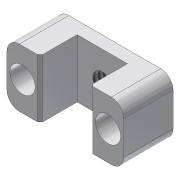
# Autodesk Inventor part: J002866
Saved by Autodesk Inventor 2012 SP2 (Build 160219200, 219)
## iProperties
Created: 2014-09-05
Material: ALUMINUM, 6061-T651
Vendor: HHMI: JFRC - ID&F
Document SubType Name: Modeling
Designer: arnoldj
Density: 2.7 g/cm^3
Part Number: J002866
Description: MPS Clamp Base
Mass: 8.49336 g
Surface Area: 23.5397 cm^2
Volume: 3.14569 cm^3
Project: P-194005
RuleStatus: InUse
AfterDocSave0: file://Part Number Cleaner
LAB/DEPT: SVOBODA (LAB)
REQUESTING SCIENTIST: PERON, SIMON
SURFACE ROUGHNESS: 63 Ra
DESIGN DEPARTMENT: HHMI: JFRC - ID&F
SPECIAL FINISH: ANODIZE PER MIL-A-8625F, TYPE II, CLASS 2 (BLACK)
ALTERED ITEM PART NUMBER: N/A
ALTERED ITEM VENDOR: N/A
ALTERED ITEM DESCRIPTION: N/A
PART NUMBER - LEGACY: J002866
Revision Number: -
Autodesk Inventor part; units mm, degrees
ref_plane "YZ Plane" through (0, 0, 0) normal (1, 0, 0) x (0, 1, 0)
ref_plane "XZ Plane" through (0, 0, 0) normal (0, 1, 0) x (-1, 0, 0)
ref_plane "XY Plane" through (0, 0, 0) normal (0, 0, 1) x (1, 0, 0)
sketch "Sketch1" plane through (0, 0, 0) normal (0, 0, 1) x (1, 0, 0)
  line L0 (-15, 7.5) -> (15, 7.5)
  line L1 (15, 7.5) -> (15, -7.5)
  line L2 (15, -7.5) -> (-15, -7.5)
  line L3 (-15, -7.5) -> (-15, 7.5)
  point P0 (0, 0)
  point P1 (-15, 0)
  point P2 (0, 7.5)
  dimension "d0" = 30
  dimension "d1" = 15
  constraints: 8 end point, 2 midpoint, 2 parallel, 1 horizontal, 1 horizontal alignment, 1 perpendicular, 1 vertical alignment
  measures "d0" distance of L0.start L0.end
  measures "d1" distance of L0.end L1.end
extrude "Extrusion1" add sketch "Sketch1" along normal blind 12.7
sketch "Sketch3" plane through (0, 0, 12.7) normal (0, 0, 1) x (1, 0, 0)
  line L0 (-15, 7.5) -> (15, 7.5) projected
  line L1 (15, -7.5) -> (-15, -7.5) projected
  line L2 (-6.477, 7.5) -> (6.477, 7.5)
  line L3 (6.477, 7.5) -> (6.477, -7.5)
  line L4 (6.477, -7.5) -> (-6.477, -7.5)
  line L5 (-6.477, -7.5) -> (-6.477, 7.5)
  point P0 (0, 0)
  point P1 (0, 7.5)
  dimension "d13" = 12.954
  constraints: 8 end point, 2 parallel, 2 point on line, 1 horizontal, 1 midpoint, 1 perpendicular, 1 vertical alignment
  measures "d13" distance of L2.start L2.end
extrude "Extrusion2" cut sketch "Sketch3" against normal blind 9.525
sketch "Sketch4" plane through (0, 0, 0) normal (0, 0, -1) x (-1, 0, 0)
  point P0 (0, 0)
  point P1 (0, 0)
  constraints: 1 coincident
hole "Hole2" at (0, 0, 0) direction (0, 0, 1) diameter 4.9784 end through all thread size "1/4-20 UNC" class "2B" standard "ANSI Unified Screw Threads"
sketch "Sketch5" plane through (0, 0, 12.7) normal (0, 0, 1) x (1, 0, 0)
  point P0 (0, 0)
  point P1 (-11, 0)
  point P2 (11, 0)
  dimension "d23" = 11
  dimension "d24" = 11
  measures "d23" distance of point (0, 0) point (11, 0)
  measures "d24" distance of point (0, 0) point (-11, 0)
hole "Hole3" at (-11, 0, 12.7) at (11, 0, 12.7) direction (0, 0, -1) diameter 3.4544 end through all counterbore diameter 6.5024 counterbore depth 6.35 clearance for "Socket Head Cap Screw" size "M3" standard "Ansi Metric M Profile"
chamfer "Chamfer1" distance 0.635 angle 45 2 edges at (6.477, 0, 12.7) (-6.477, 0, 12.7)
fillet "Fillet1" radius 3.175 4 edges at (15, 7.5, 6.35) (-15, 7.5, 6.35) (-15, -7.5, 6.35) (15, -7.5, 6.35)
body "Solid1"
